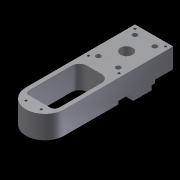
# Autodesk Inventor part: JointC3'_2nd
Saved by Autodesk Inventor 2011 SP1 (Build 150282100, 282)
## iProperties
Created: 2013-02-06
Part Number: JointC3'_2nd
Document SubType Name: Modeling
Designer: arihon
Density: 1 g/cm^3
Author: arihon
Autodesk Inventor part; units mm, degrees
ref_plane "YZ Plane" through (0, 0, 0) normal (1, 0, 0) x (0, 1, 0)
ref_plane "XZ Plane" through (0, 0, 0) normal (0, 1, 0) x (-1, 0, 0)
ref_plane "XY Plane" through (0, 0, 0) normal (0, 0, 1) x (1, 0, 0)
sketch "スケッチ1" plane through (0, 0, 0) normal (0, 0, 1) x (1, 0, 0)
  line L0 (-12.5, 36) -> (12.5, 36)
  line L1 (12.5, 36) -> (12.5, -48)
  line L2 (12.5, -48) -> (-12.5, -48)
  line L3 (-12.5, -48) -> (-12.5, 36)
  point P0 (0, 0)
  dimension "d0" = 36
  dimension "d1" = 25
  dimension "d2" = 12.5
  dimension "d3" = 48
  constraints: 8 end point, 2 parallel, 1 horizontal, 1 perpendicular
  measures "d0" distance from line of point (0, 0) L0
  measures "d1" distance between parallel lines of L1 L3
  measures "d2" distance from line of L1 point (0, 0)
  measures "d3" distance from line of L2 point (0, 0)
extrude "押し出し1" add sketch "スケッチ1" along normal blind 15
sketch "スケッチ2" plane through (0, 0, 0) normal (0, 0, -1) x (-1, 0, 0)
  line L0 (-12.5, 36) -> (-12.5, -48) projected
  line L1 (12.5, -48) -> (12.5, 36) projected
  line L2 (-12.5, 36) -> (12.5, 36)
  line L3 (12.5, 36) -> (12.5, 24)
  line L4 (12.5, 24) -> (-12.5, 24)
  line L5 (-12.5, 24) -> (-12.5, 36)
  line L6 (12.5, 0) -> (-12.5, 0)
  line L7 (-12.5, 0) -> (-12.5, 12)
  line L8 (-12.5, 12) -> (12.5, 12)
  line L9 (12.5, 12) -> (12.5, 0)
  point P0 (0, 0)
  dimension "d6" = 12
  dimension "d42" = 12
  dimension "d66" = 12
  constraints: 16 end point, 4 parallel, 2 horizontal, 2 perpendicular, 2 point on line
  measures "d6" distance between parallel lines of L4 L2
  measures "d42" distance between parallel lines of L6 L8
  measures "d66" distance between parallel lines of L8 L4
extrude "押し出し2" cut sketch "スケッチ2" against normal blind 2 contours L2 L1 L4 L0 | L8 L1 L6 L0
sketch "スケッチ3" plane through (0, 0, 2) normal (0, 0, -1) x (-1, 0, 0)
  line L0 (12.5, 36) -> (12.5, 24) projected
  line L1 (-12.5, 36) -> (12.5, 36) projected
  line L2 (-12.5, 24) -> (-12.5, 36) projected
  point P0 (0, 0)
  point P1 (-6.5, 30)
  point P2 (6.5, 30)
  point P3 (12.5, 0)
  point P4 (-12.5, 0)
  dimension "d10" = 6
  dimension "d11" = 6
  dimension "d12" = 6
  dimension "d13" = 6
  measures "d10" distance from line of L2 point (-6.5, 30)
  measures "d11" distance from line of L0 point (6.5, 30)
  measures "d12" distance from line of point (-6.5, 30) L1
  measures "d13" distance from line of L1 point (6.5, 30)
hole "Hole1" at (6.5, 30, 2) at (-6.5, 30, 2) direction (0, 0, 1) diameter 3.242 end through all thread size "M4x0.7" class "6H" standard "ISO Metric profile"
sketch "スケッチ6" plane through (0, 0, 2) normal (0, 0, -1) x (-1, 0, 0)
  line L0 (-12.5, 0) -> (12.5, 0) projected
  line L1 (12.5, 12) -> (12.5, 0) projected
  line L2 (-12.5, 0) -> (-12.5, 12) projected
  point P0 (0, 0)
  point P1 (-6.5, 6)
  point P2 (6.5, 6)
  dimension "d43" = 6
  dimension "d44" = 6
  dimension "d45" = 6
  dimension "d46" = 6
  measures "d43" distance from line of L0 point (-6.5, 6)
  measures "d44" distance from line of L0 point (6.5, 6)
  measures "d45" distance from line of L2 point (-6.5, 6)
  measures "d46" distance from line of L1 point (6.5, 6)
hole "Hole4" at (6.5, 6, 2) at (-6.5, 6, 2) direction (0, 0, 1) diameter 3.242 end through all thread size "M4x0.7" class "6H" standard "ANSI Metric M Profile"
sketch "スケッチ7" plane through (0, 0, 0) normal (0, 0, -1) x (-1, 0, 0)
  line L0 (12.5, 24) -> (-12.5, 24) projected
  line L1 (12.5, 12) -> (12.5, 24) projected
  point P0 (0, 0)
  point P1 (0, 18)
  dimension "d54" = 6
  dimension "d55" = 12.5
  measures "d54" distance from line of point (0, 18) L0
  measures "d55" distance from line of L1 point (0, 18)
hole "Hole5" at (0, 18, 0) direction (0, 0, 1) diameter 8 end through all
sketch "スケッチ8" plane through (0, 0, 0) normal (0, 0, -1) x (-1, 0, 0)
  line L0 (12.5, 0) -> (-12.5, 0) projected
  line L1 (-12.5, 0) -> (-12.5, -48) projected
  line L2 (-12.5, -48) -> (12.5, -48) projected
  line L3 (12.5, -48) -> (12.5, 0) projected
  line L4 (0, 0) -> (0, -48)
  line L5 (12.5, -24) -> (-12.5, -24)
  line L6 (-9.85, -3.15) -> (9.85, -3.15)
  line L7 (9.85, -3.15) -> (9.85, -39.05)
  line L8 (9.85, -39.05) -> (-9.85, -39.05)
  line L9 (-9.85, -39.05) -> (-9.85, -3.15)
  dimension "d63" = 19.7
  dimension "d64" = 19.7
  dimension "d65" = 35.9
  dimension "d68" = 3.15
  constraints: 12 end point, 3 midpoint, 2 parallel, 1 horizontal, 1 perpendicular
  measures "d63" distance of L6.start L6.end
  measures "d64" diameter of L7 L4
  measures "d65" distance of L6.end L7.end
  measures "d68" distance between parallel lines of L6 L0
extrude "押し出し3" cut sketch "スケッチ8" against normal through all contours L6 L7 L5 L4 | L4 L5 L9 L6 | L7 L8 L4 L5 | L4 L8 L9 L5
fillet "フィレット2" radius 5.05 2 edges at (9.85, -3.15, 7.5) (-9.85, -3.15, 7.5)
fillet "フィレット3" radius 3.05 2 edges at (9.85, -39.05, 7.5) (-9.85, -39.05, 7.5)
fillet "フィレット4" radius 12.5 2 edges at (12.5, -48, 7.5) (-12.5, -48, 7.5)
sketch "スケッチ13" plane through (0, 0, 15) normal (0, 0, 1) x (1, 0, 0)
  arc A0 (-12.5, -35.5) -> (12.5, -35.5) centre (0, -35.5) ccw projected
  line L0 (12.5, 36) -> (12.5, -35.5) projected
  line L1 (-12.5, 36) -> (12.5, 36) projected
  line L2 (-12.5, -35.5) -> (-12.5, 36) projected
  circle A1 centre (-6.5, 6) radius 1.621 projected
  circle A2 centre (6.5, 6) radius 1.621 projected
  point P0 (0, 0)
  point P1 (-10, 33.5)
  point P2 (10, 33.5)
  point P3 (-10, 3)
  point P4 (10, 3)
  point P5 (-5, -43)
  point P6 (5, -43)
  dimension "d106" = 2.5
  dimension "d107" = 2.5
  dimension "d108" = 2.5
  dimension "d109" = 2.5
  dimension "d110" = 2.5
  dimension "d111" = 2.5
  dimension "d112" = 3
  dimension "d113" = 3
  dimension "d114" = 5
  dimension "d115" = 5
  dimension "d125" = 79
  dimension "d126" = 79
  measures "d106" distance from line of point (-10, 33.5) L1
  measures "d107" distance from line of L2 point (-10, 33.5)
  measures "d108" distance from line of L0 point (10, 33.5)
  measures "d109" distance from line of point (10, 33.5) L1
  measures "d110" distance from line of L2 point (-10, 3)
  measures "d111" distance from line of L0 point (10, 3)
  measures "d112" vertical distance of point (-10, 3) A1.centre
  measures "d113" vertical distance of point (10, 3) A2.centre
  measures "d114" horizontal distance of A0.centre point (-5, -43)
  measures "d115" horizontal distance of point (5, -43) A0.centre
  measures "d125" distance from line of point (5, -43) L1
  measures "d126" distance from line of point (-5, -43) L1
hole "Hole8" at (-10, 33.5, 15) at (10, 33.5, 15) at (-10, 3, 15) at (10, 3, 15) at (-5, -43, 15) at (5, -43, 15) direction (0, 0, -1) diameter 1.567 end through all thread size "M2x0.4" class "6H" standard "ISO Metric profile"
sketch "スケッチ14" plane through (0, 0, 0) normal (0, 0, -1) x (-1, 0, 0)
  circle A0 centre (0, 18) radius 4 projected
  line L0 (12.5, 24) -> (-12.5, 24) projected
  line L1 (-12.5, 24) -> (-12.5, 12) projected
  line L2 (-12.5, 12) -> (12.5, 12) projected
  line L3 (12.5, 12) -> (12.5, 24) projected
  line L4 (-10.4, 24) -> (10.4, 24)
  line L5 (10.4, 24) -> (10.4, 12)
  line L6 (10.4, 12) -> (-10.4, 12)
  line L7 (-10.4, 12) -> (-10.4, 24)
  point P0 (0, 0)
  dimension "d127" = 2.1
  dimension "d128" = 2.1
  constraints: 8 end point, 2 parallel, 2 point on line, 1 horizontal, 1 perpendicular
  measures "d127" distance between parallel lines of L1 L7
  measures "d128" distance between parallel lines of L5 L3
extrude "押し出し4" add sketch "スケッチ14" along normal blind 5 contours L5 L2 L7 L0
equation "\"d2\" = 0.5 * d1"
equation "\"d42\" = d6"
equation "\"d66\" = d42"
equation "\"d10\" = d12"
equation "\"d11\" = d10"
equation "\"d13\" = d12"
equation "\"d44\" = d43"
equation "\"d45\" = d43"
equation "\"d46\" = d43"
equation "\"d64\" = d63"
equation "\"d107\" = d106"
equation "\"d108\" = d106"
equation "\"d109\" = d106"
equation "\"d110\" = d106"
equation "\"d111\" = d106"
equation "\"d115\" = d114"
equation "\"d126\" = d125"
equation "\"d128\" = d127"
